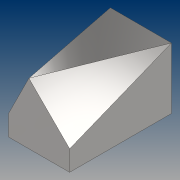
# Autodesk Inventor part: 40
Saved by Autodesk Inventor 2020.2 (Build 242310000, 310)
## iProperties
Created: 2020-09-17
Part Number: 40
Material: 鋼、碳鋼
Document SubType Name: Modeling
Designer: user
Density: 7.85 g/cm^3
Appearance: 半拋光
Mass: 314 g
Surface Area: 70.5274 cm^2
Volume: 40 cm^3
Author: user
Autodesk Inventor part; units mm, degrees
ref_plane "YZ Plane" through (0, 0, 0) normal (1, 0, 0) x (0, 1, 0)
ref_plane "XZ Plane" through (0, 0, 0) normal (0, 1, 0) x (-1, 0, 0)
ref_plane "XY Plane" through (0, 0, 0) normal (0, 0, 1) x (1, 0, 0)
sketch "草圖1" plane through (0, 0, 0) normal (0, 1, 0) x (-1, 0, 0)
  line L0 (15, 0) -> (-15, 0)
  line L1 (-15, 0) -> (-15, 50)
  line L2 (-15, 50) -> (15, 50)
  line L3 (15, 50) -> (15, 0)
  point P0 (0, 0)
  point P1 (0, 0)
  dimension "d0" = 30
  dimension "d1" = 50
  constraints: 8 end point, 2 parallel, 1 coincident, 1 horizontal, 1 midpoint, 1 perpendicular
  measures "d0" distance of L1.end L2.end
  measures "d1" distance of L2.end L0.start
extrude "擠出1" add sketch "草圖1" along normal blind 30
sketch "草圖2" plane through (-15, 0, 50) normal (0, 0, 1) x (1, 0, 0)
  line L0 (0, 0) -> (0, 30) construction
  line L1 (0, 30) -> (30, 30) construction
  line L2 (30, 30) -> (30, 0) construction
  line L3 (30, 0) -> (0, 0) construction
  line L4 (0, 0) -> (0, 30) construction
  line L5 (0, 10) -> (10, 30)
  line L6 (0, 30) -> (30, 30) construction
  line L7 (10, 30) -> (0, 30)
  line L8 (0, 30) -> (0, 10)
  point P0 (15, 0)
  dimension "d4" = 10
  dimension "d5" = 20
  constraints: 6 end point, 2 collinear, 2 point on line
  measures "d4" distance from line of L5.end L0
  measures "d5" distance from line of L5.start L1
loft "斷面混成1" cut profiles "草圖2" section 2 point at (-15, 30, 0)
sketch "草圖3" plane through (-15, 0, 50) normal (0, 0, 1) x (1, 0, 0)
  line L0 (0, 10) -> (10, 30) construction
  line L1 (10, 30) -> (30, 30) construction
  line L2 (30, 30) -> (30, 0) construction
  line L3 (30, 0) -> (0, 0) construction
  line L4 (0, 0) -> (0, 10) construction
  line L5 (10, 30) -> (30, 10)
  line L6 (30, 30) -> (0, 30) construction
  line L7 (30, 10) -> (30, 30)
  line L8 (30, 30) -> (10, 30)
  point P0 (15, 0)
  dimension "d10" = 20
  constraints: 6 end point, 1 collinear, 1 perpendicular, 1 point on line
  measures "d10" distance from line of L1 L5.end
loft "斷面混成2" cut profiles "草圖3" section 2 point at (15, 30, 0)
